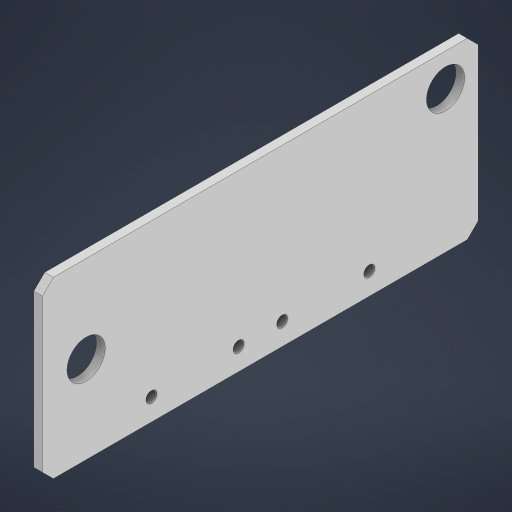
# Autodesk Inventor part: ArmSidePlateInner
Saved by Autodesk Inventor 2024 (Build 280153000, 153)
## iProperties
Created: 2023-10-25
Part Number: ArmSidePlateInner
Material: Generic
Document SubType Name: Modeling
Designer: avsar
Density: 1 g/cm^3
Appearance: Default
Author: avsar
Autodesk Inventor part; units mm, degrees
ref_plane "YZ Plane" through (0, 0, 0) normal (1, 0, 0) x (0, 1, 0)
ref_plane "XZ Plane" through (0, 0, 0) normal (0, 1, 0) x (-1, 0, 0)
ref_plane "XY Plane" through (0, 0, 0) normal (0, 0, 1) x (1, 0, 0)
sketch "Sketch1" plane through (0, 0, 0) normal (1, 0, 0) x (0, 1, 0)
  line L0 (-32, 80) -> (32, 80)
  line L1 (32, 80) -> (32, -80)
  line L2 (32, -80) -> (-32, -80)
  line L3 (-32, -80) -> (-32, 80)
  line L4 (-32, 80) -> (32, -80) construction
  line L5 (32, 80) -> (-32, -80) construction
  point P0 (0, 0)
  dimension "d0" = 64
  dimension "d1" = 160
  constraints: 12 end point, 2 midpoint, 2 parallel, 1 horizontal, 1 perpendicular
  measures "d0" distance of L1.end L2.end
  measures "d1" distance of L0.end L1.end
extrude "Extrusion1" add sketch "Sketch1" along normal blind 3.175
chamfer "Chamfer1" distance 4 angle 45 2 edges at (1.5875, 32, 80) (1.5875, 32, -80)
chamfer "Chamfer2" distance 4 angle 45 2 edges at (1.5875, -32, 80) (1.5875, -32, -80)
sketch "Sketch3" plane through (3.175, 0, 0) normal (1, 0, 0) x (0, 0, -1)
  circle A0 centre (-24, -8) radius 7 construction
  circle A1 centre (-8, -24) radius 2
  line L0 (-76, -32) -> (76, -32) construction
  line L1 (-24, -1) -> (-24, -15) construction
  circle A2 centre (-40, -24) radius 2
  line L2 (76, 32) -> (-76, 32) construction
  line L3 (0, 32) -> (0, -32) construction
  circle A3 centre (8, -24) radius 2
  circle A4 centre (40, -24) radius 2
  point P0 (0, 0)
  dimension "d3" = 0
  dimension "d22" = 14
  dimension "d23" = 24
  dimension "d24" = 4
  dimension "d25" = 16
  dimension "d26" = 8
  dimension "d27" = 16
  constraints: 5 centre point, 4 end point, 3 midpoint, 3 symmetric about line, 2 point on circle, 1 coincident, 1 vertical, 3 other
  measures "d22" diameter of A0
  measures "d23" horizontal distance of point (0, 0) A0.centre
  measures "d24" diameter of A1
  measures "d25" horizontal distance of A1.centre A0.centre
  measures "d26" distance from line of L0 A1.centre
  measures "d27" horizontal distance of A1.centre A0.centre
extrude "Extrusion3" cut sketch "Sketch3" against normal through all
sketch "Sketch4" plane through (3.175, 0, 0) normal (1, 0, 0) x (0, 0, -1)
  circle A0 centre (-64, 0) radius 7
  point P0 (0, 0)
  dimension "d30" = 14
  dimension "d31" = 64
  constraints: 1 centre point, 1 horizontal alignment
  measures "d30" diameter of A0
  measures "d31" distance of point (0, 0) A0.centre
extrude "Extrusion4" cut sketch "Sketch4" against normal through all
sketch "Sketch6" plane through (3.175, 0, 0) normal (1, 0, 0) x (0, 0, -1)
  circle A0 centre (-64, 0) radius 7 construction
  circle A1 centre (68, 20) radius 7
  line L0 (68, 20) -> (75, 20) construction
  point P0 (0, 0)
  dimension "d65" = 14
  dimension "d67" = 68
  dimension "d68" = 20
  constraints: 2 end point, 1 horizontal, 1 horizontal alignment, 2 other
  measures "d67" horizontal distance of L0.start point (0, 0)
  measures "d68" vertical distance of point (0, 0) L0.start
extrude "Extrusion6" cut sketch "Sketch6" against normal blind 10
body "Solid1"
